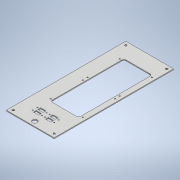
# Autodesk Inventor part: top_panel2
Saved by Autodesk Inventor 2022 (Build 260153000, 153)
## iProperties
Created: 2021-05-16
Part Number: top_panel2
Material: Generic
Document SubType Name: Modeling
Designer: gisen
Density: 1 g/cm^3
Appearance: Default
Author: gisen
Autodesk Inventor part; units mm, degrees
ref_plane "YZ Plane" through (0, 0, 0) normal (1, 0, 0) x (0, 1, 0)
ref_plane "XZ Plane" through (0, 0, 0) normal (0, 1, 0) x (-1, 0, 0)
ref_plane "XY Plane" through (0, 0, 0) normal (0, 0, 1) x (1, 0, 0)
sketch "Sketch1" plane through (0, 0, 0) normal (0, 0, 1) x (1, 0, 0)
  line L0 (-78, 195) -> (78, 195)
  line L1 (78, 195) -> (78, -195)
  line L2 (78, -195) -> (-78, -195)
  line L3 (-78, -195) -> (-78, 195)
  line L4 (-78, 195) -> (78, -195) construction
  line L5 (78, 195) -> (-78, -195) construction
  point P0 (0, 0)
  dimension "d1" = 156
  dimension "d2" = 390
  constraints: 12 end point, 2 midpoint, 2 parallel, 1 horizontal, 1 perpendicular
  measures "d1" distance of L0.start L0.end
  measures "d2" distance of L0.end L1.end
extrude "Extrusion1" add sketch "Sketch1" along normal blind 3
sketch "Sketch2" plane through (0, 0, 3) normal (0, 0, 1) x (1, 0, 0)
  line L0 (-78, -195) -> (78, -195) projected
  line L1 (-78, 195) -> (-78, -195) projected
  arc A0 (-64.4298, -185.2577) -> (-68.2577, -181.4298) centre (-66, -183) ccw
  arc A1 (-69.8472, -183.7153) -> (-66.7153, -186.8472) centre (-68, -185) ccw
  line L2 (-66.7153, -186.8472) -> (-64.4298, -185.2577)
  line L3 (-69.8472, -183.7153) -> (-68.2577, -181.4298)
  line L4 (0, 16.0888) -> (0, -25.3045)
  line L5 (-19.6832, 0) -> (22.709, 0)
  arc A2 (68.2577, -181.4298) -> (64.4298, -185.2577) centre (66, -183) ccw
  arc A3 (66.7153, -186.8472) -> (69.8472, -183.7153) centre (68, -185) ccw
  line L6 (66.7153, -186.8472) -> (64.4298, -185.2577)
  line L7 (69.8472, -183.7153) -> (68.2577, -181.4298)
  arc A4 (-68.2577, 181.4298) -> (-64.4298, 185.2577) centre (-66, 183) ccw
  arc A5 (-66.7153, 186.8472) -> (-69.8472, 183.7153) centre (-68, 185) ccw
  line L8 (-66.7153, 186.8472) -> (-64.4298, 185.2577)
  line L9 (-69.8472, 183.7153) -> (-68.2577, 181.4298)
  arc A6 (64.4298, 185.2577) -> (68.2577, 181.4298) centre (66, 183) ccw
  arc A7 (69.8472, 183.7153) -> (66.7153, 186.8472) centre (68, 185) ccw
  line L10 (66.7153, 186.8472) -> (64.4298, 185.2577)
  line L11 (69.8472, 183.7153) -> (68.2577, 181.4298)
  point P0 (0, 0)
  dimension "d11" = 12
  dimension "d12" = 10
  dimension "d13" = 12
  dimension "d14" = 10
  dimension "d15" = 5.5
  dimension "d16" = 4.5
  constraints: 24 symmetric about line, 20 end point, 16 point on circle, 8 centre point, 8 coincident, 4 tangent, 1 horizontal, 1 vertical, 6 other
  measures "d11" distance from line of L0 point (-66, -183)
  measures "d12" distance from line of L0 point (-68, -185)
  measures "d13" distance from line of L1 point (-66, -183)
  measures "d14" distance from line of L1 point (-68, -185)
  measures "d15" diameter of A0
  measures "d16" diameter of A1
extrude "Extrusion2" cut sketch "Sketch2" against normal up to surface (3 mm away)
sketch "Sketch4" plane through (0, 0, 3) normal (0, 0, 1) x (1, 0, 0)
  line L0 (-28.5, -132.4667) -> (-11.5, -132.4667)
  line L1 (-11.5, -132.4667) -> (-11.5, -141.4667)
  line L2 (-11.5, -141.4667) -> (-28.5, -141.4667)
  line L3 (-28.5, -141.4667) -> (-28.5, -132.4667)
  line L4 (-28.5, -132.4667) -> (-11.5, -141.4667) construction
  line L5 (-11.5, -132.4667) -> (-28.5, -141.4667) construction
  circle A0 centre (-35, -136.9667) radius 1.65
  circle A1 centre (-5, -136.9667) radius 1.65
  line L6 (0, -132.1595) -> (0, -155.449)
  line L7 (28.5, -132.4667) -> (11.5, -132.4667)
  line L8 (11.5, -132.4667) -> (11.5, -141.4667)
  line L9 (11.5, -141.4667) -> (28.5, -141.4667)
  line L10 (28.5, -141.4667) -> (28.5, -132.4667)
  line L11 (28.5, -132.4667) -> (11.5, -141.4667) construction
  line L12 (11.5, -132.4667) -> (28.5, -141.4667) construction
  circle A2 centre (35, -136.9667) radius 1.65
  circle A3 centre (5, -136.9667) radius 1.65
  line L13 (-30.7879, -144.4667) -> (-3.35, -144.4667)
  line L14 (-28.5, -156.4667) -> (-11.5, -156.4667)
  line L15 (-11.5, -156.4667) -> (-11.5, -147.4667)
  line L16 (-11.5, -147.4667) -> (-28.5, -147.4667)
  line L17 (-28.5, -147.4667) -> (-28.5, -156.4667)
  line L18 (-28.5, -156.4667) -> (-11.5, -147.4667) construction
  line L19 (-11.5, -156.4667) -> (-28.5, -147.4667) construction
  circle A4 centre (-35, -151.9667) radius 1.65
  circle A5 centre (-5, -151.9667) radius 1.65
  line L20 (28.5, -156.4667) -> (11.5, -156.4667)
  line L21 (11.5, -156.4667) -> (11.5, -147.4667)
  line L22 (11.5, -147.4667) -> (28.5, -147.4667)
  line L23 (28.5, -147.4667) -> (28.5, -156.4667)
  line L24 (28.5, -156.4667) -> (11.5, -147.4667) construction
  line L25 (11.5, -156.4667) -> (28.5, -147.4667) construction
  circle A6 centre (35, -151.9667) radius 1.65
  circle A7 centre (5, -151.9667) radius 1.65
  line L26 (-66.7153, 186.8472) -> (-64.4298, 185.2577) projected
  arc A8 (-68.2577, 181.4298) -> (-64.4298, 185.2577) centre (-66, 183) ccw projected
  line L27 (-68.2577, 181.4298) -> (-69.8472, 183.7153) projected
  arc A9 (-66.7153, 186.8472) -> (-69.8472, 183.7153) centre (-68, 185) ccw projected
  arc A10 (69.8472, 183.7153) -> (66.7153, 186.8472) centre (68, 185) ccw projected
  line L28 (69.8472, 183.7153) -> (68.2577, 181.4298) projected
  arc A11 (64.4298, 185.2577) -> (68.2577, 181.4298) centre (66, 183) ccw projected
  line L29 (64.4298, 185.2577) -> (66.7153, 186.8472) projected
  line L30 (66.7153, -186.8472) -> (64.4298, -185.2577) projected
  arc A12 (68.2577, -181.4298) -> (64.4298, -185.2577) centre (66, -183) ccw projected
  line L31 (68.2577, -181.4298) -> (69.8472, -183.7153) projected
  arc A13 (66.7153, -186.8472) -> (69.8472, -183.7153) centre (68, -185) ccw projected
  arc A14 (-69.8472, -183.7153) -> (-66.7153, -186.8472) centre (-68, -185) ccw projected
  line L32 (-69.8472, -183.7153) -> (-68.2577, -181.4298) projected
  arc A15 (-64.4298, -185.2577) -> (-68.2577, -181.4298) centre (-66, -183) ccw projected
  line L33 (-64.4298, -185.2577) -> (-66.7153, -186.8472) projected
  line L34 (78, 195) -> (-78, 195) projected
  line L35 (-78, 195) -> (-78, -195) projected
  line L36 (-78, -195) -> (78, -195) projected
  line L37 (78, -195) -> (78, 195) projected
  line L38 (78, -195) -> (-78, -195) projected
  point P0 (0, 0)
  point P1 (-20, -136.9667)
  point P2 (-5, -136.9667)
  point P3 (20, -136.9667)
  point P4 (-20, -151.9667)
  point P5 (20, -151.9667)
  point P6 (0, -195)
  dimension "d37" = 17
  dimension "d38" = 9
  dimension "d39" = 6.5
  dimension "d40" = 4.5
  dimension "d41" = 3.3
  dimension "d42" = 6.5
  dimension "d43" = 4.5
  dimension "d44" = 3.3
  dimension "d45" = 5
  dimension "d46" = 3
  dimension "d55" = 0
  constraints: 52 end point, 27 symmetric about line, 9 midpoint, 8 centre point, 8 coincident, 2 horizontal, 2 parallel, 1 perpendicular, 1 vertical, 6 other
  measures "d37" distance of L1.end L2.end
  measures "d38" distance of L0.end L1.end
  measures "d39" distance from line of L3 point (-35, -136.967)
  measures "d40" distance from line of point (-35, -136.967) L0
  measures "d41" diameter of A0
  measures "d42" distance from line of point (-5, -136.967) L1
  measures "d43" distance from line of L0 point (-5, -136.967)
  measures "d44" diameter of A1
  measures "d45" horizontal distance of A1.centre point (0, 0)
  measures "d46" distance between parallel lines of L13 L2
  measures "d55" distance from line of point (0, -195) L6
extrude "Extrusion4" cut sketch "Sketch4" against normal up to surface (3 mm away) contours L0 L1 L2 L3 | A0 | A1 | L10 L9 L8 L7 | A2 | A3 | L17 L16 L15 L14 | A4 | A5 | L20 L21 L22 L23 | A6 | A7
sketch "Sketch5" plane through (0, 0, 3) normal (0, 0, 1) x (1, 0, 0)
  line L0 (-78, -195) -> (78, -195) projected
  line L1 (-2.4755, -172.54) -> (2.4755, -172.54)
  line L2 (-2.4755, -187.46) -> (2.4755, -187.46)
  arc A0 (-2.4755, -172.54) -> (-2.4755, -187.46) centre (0, -180) ccw
  arc A1 (2.4755, -187.46) -> (2.4755, -172.54) centre (0, -180) ccw
  point P0 (0, 0)
  dimension "d49" = 15
  dimension "d51" = 7.46
  dimension "d52" = 7.46
  constraints: 4 end point, 4 point on circle, 2 centre point, 2 horizontal, 1 coincident
  measures "d49" distance from line of L0 point (0, -180)
  measures "d51" distance from line of A0.centre L1
  measures "d52" distance from line of point (0, -180) L2
extrude "Extrusion5" cut sketch "Sketch5" against normal up to surface (3 mm away)
sketch "Sketch7" plane through (0, 0, 3) normal (0, 0, 1) x (1, 0, 0)
  circle A0 centre (-38, -90.5) radius 2
  line L0 (-2.4755, -172.54) -> (2.4755, -172.54) projected
  arc A1 (2.4755, -187.46) -> (2.4755, -172.54) centre (0, -180) ccw projected
  line L1 (2.4755, -187.46) -> (-2.4755, -187.46) projected
  arc A2 (-2.4755, -172.54) -> (-2.4755, -187.46) centre (0, -180) ccw projected
  line L2 (-11.5, -156.4667) -> (-28.5, -156.4667) projected
  line L3 (-28.5, -156.4667) -> (-28.5, -147.4667) projected
  line L4 (-28.5, -147.4667) -> (-11.5, -147.4667) projected
  line L5 (-11.5, -147.4667) -> (-11.5, -156.4667) projected
  line L6 (11.5, -147.4667) -> (28.5, -147.4667) projected
  line L7 (28.5, -147.4667) -> (28.5, -156.4667) projected
  line L8 (28.5, -156.4667) -> (11.5, -156.4667) projected
  line L9 (11.5, -156.4667) -> (11.5, -147.4667) projected
  line L10 (11.5, -132.4667) -> (28.5, -132.4667) projected
  line L11 (28.5, -132.4667) -> (28.5, -141.4667) projected
  line L12 (28.5, -141.4667) -> (11.5, -141.4667) projected
  line L13 (11.5, -141.4667) -> (11.5, -132.4667) projected
  circle A3 centre (35, -151.9667) radius 1.65 projected
  circle A4 centre (-35, -151.9667) radius 1.65 projected
  circle A5 centre (5, -136.9667) radius 1.65 projected
  circle A6 centre (-5, -136.9667) radius 1.65 projected
  circle A7 centre (-35, -136.9667) radius 1.65 projected
  circle A8 centre (35, -136.9667) radius 1.65 projected
  circle A9 centre (-5, -151.9667) radius 1.65 projected
  circle A10 centre (5, -151.9667) radius 1.65 projected
  line L14 (-11.5, -132.4667) -> (-11.5, -141.4667) projected
  line L15 (-11.5, -141.4667) -> (-28.5, -141.4667) projected
  line L16 (-28.5, -141.4667) -> (-28.5, -132.4667) projected
  line L17 (-28.5, -132.4667) -> (-11.5, -132.4667) projected
  line L18 (-66.7153, 186.8472) -> (-64.4298, 185.2577) projected
  arc A11 (-68.2577, 181.4298) -> (-64.4298, 185.2577) centre (-66, 183) ccw projected
  line L19 (-68.2577, 181.4298) -> (-69.8472, 183.7153) projected
  arc A12 (-66.7153, 186.8472) -> (-69.8472, 183.7153) centre (-68, 185) ccw projected
  arc A13 (69.8472, 183.7153) -> (66.7153, 186.8472) centre (68, 185) ccw projected
  line L20 (69.8472, 183.7153) -> (68.2577, 181.4298) projected
  arc A14 (64.4298, 185.2577) -> (68.2577, 181.4298) centre (66, 183) ccw projected
  line L21 (64.4298, 185.2577) -> (66.7153, 186.8472) projected
  line L22 (66.7153, -186.8472) -> (64.4298, -185.2577) projected
  arc A15 (68.2577, -181.4298) -> (64.4298, -185.2577) centre (66, -183) ccw projected
  line L23 (68.2577, -181.4298) -> (69.8472, -183.7153) projected
  arc A16 (66.7153, -186.8472) -> (69.8472, -183.7153) centre (68, -185) ccw projected
  arc A17 (-69.8472, -183.7153) -> (-66.7153, -186.8472) centre (-68, -185) ccw projected
  line L24 (-69.8472, -183.7153) -> (-68.2577, -181.4298) projected
  arc A18 (-64.4298, -185.2577) -> (-68.2577, -181.4298) centre (-66, -183) ccw projected
  line L25 (-64.4298, -185.2577) -> (-66.7153, -186.8472) projected
  line L26 (78, 195) -> (-78, 195) projected
  line L27 (-78, 195) -> (-78, -195) projected
  line L28 (-78, -195) -> (78, -195) projected
  line L29 (78, -195) -> (78, 195) projected
  circle A19 centre (-38, 14.5) radius 2
  circle A20 centre (-38, 30) radius 2
  circle A21 centre (-38, 135) radius 2
  line L30 (14.5, 19.3358) -> (14.5, -21.6)
  circle A22 centre (67, -90.5) radius 2
  circle A23 centre (67, 14.5) radius 2
  circle A24 centre (67, 30) radius 2
  circle A25 centre (67, 135) radius 2
  point P0 (0, 0)
  dimension "d56" = 4
  dimension "d57" = 40
  dimension "d60" = 4
  dimension "d61" = 105
  dimension "d62" = 40
  dimension "d63" = 4
  dimension "d65" = 40
  dimension "d66" = 4
  dimension "d68" = 40
  dimension "d69" = 60
  dimension "d103" = 15.5
  dimension "d104" = 105
  dimension "d112" = 52.5
  constraints: 8 centre point, 4 symmetric about line, 2 end point, 1 vertical, 4 other
  measures "d56" diameter of A0
  measures "d57" distance from line of L27 A0.centre
  measures "d60" diameter of A19
  measures "d61" distance of A0.centre A19.centre
  measures "d62" distance from line of L27 A19.centre
  measures "d63" diameter of A20
  measures "d65" distance from line of L27 A20.centre
  measures "d66" diameter of A21
  measures "d68" distance from line of L27 A21.centre
  measures "d69" distance from line of L26 A21.centre
  measures "d103" distance of A19.centre A20.centre
  measures "d104" distance of A21.centre A20.centre
  measures "d112" distance from line of A19.centre L30
extrude "Extrusion7" cut sketch "Sketch7" against normal up to surface (3 mm away) contours A0 | A19 | A20 | A21 | A22 | A23 | A24 | A25
sketch "Sketch8" plane through (0, 0, 3) normal (0, 0, 1) x (1, 0, 0)
  circle A0 centre (-38, -90.5) radius 2 projected
  circle A1 centre (-38, 14.5) radius 2 projected
  circle A2 centre (67, 30) radius 2 projected
  circle A3 centre (67, 135) radius 2 projected
  circle A4 centre (67, -90.5) radius 2 projected
  circle A5 centre (67, 14.5) radius 2 projected
  circle A6 centre (-38, 30) radius 2 projected
  circle A7 centre (-38, 135) radius 2 projected
  line L0 (-2.4755, -172.54) -> (2.4755, -172.54) projected
  arc A8 (2.4755, -187.46) -> (2.4755, -172.54) centre (0, -180) ccw projected
  line L1 (2.4755, -187.46) -> (-2.4755, -187.46) projected
  arc A9 (-2.4755, -172.54) -> (-2.4755, -187.46) centre (0, -180) ccw projected
  line L2 (-11.5, -156.4667) -> (-28.5, -156.4667) projected
  line L3 (-28.5, -156.4667) -> (-28.5, -147.4667) projected
  line L4 (-28.5, -147.4667) -> (-11.5, -147.4667) projected
  line L5 (-11.5, -147.4667) -> (-11.5, -156.4667) projected
  line L6 (11.5, -147.4667) -> (28.5, -147.4667) projected
  line L7 (28.5, -147.4667) -> (28.5, -156.4667) projected
  line L8 (28.5, -156.4667) -> (11.5, -156.4667) projected
  line L9 (11.5, -156.4667) -> (11.5, -147.4667) projected
  line L10 (11.5, -132.4667) -> (28.5, -132.4667) projected
  line L11 (28.5, -132.4667) -> (28.5, -141.4667) projected
  line L12 (28.5, -141.4667) -> (11.5, -141.4667) projected
  line L13 (11.5, -141.4667) -> (11.5, -132.4667) projected
  circle A10 centre (35, -151.9667) radius 1.65 projected
  circle A11 centre (-35, -151.9667) radius 1.65 projected
  circle A12 centre (5, -136.9667) radius 1.65 projected
  circle A13 centre (-5, -136.9667) radius 1.65 projected
  circle A14 centre (-35, -136.9667) radius 1.65 projected
  circle A15 centre (35, -136.9667) radius 1.65 projected
  circle A16 centre (-5, -151.9667) radius 1.65 projected
  circle A17 centre (5, -151.9667) radius 1.65 projected
  line L14 (-11.5, -132.4667) -> (-11.5, -141.4667) projected
  line L15 (-11.5, -141.4667) -> (-28.5, -141.4667) projected
  line L16 (-28.5, -141.4667) -> (-28.5, -132.4667) projected
  line L17 (-28.5, -132.4667) -> (-11.5, -132.4667) projected
  line L18 (-66.7153, 186.8472) -> (-64.4298, 185.2577) projected
  arc A18 (-68.2577, 181.4298) -> (-64.4298, 185.2577) centre (-66, 183) ccw projected
  line L19 (-68.2577, 181.4298) -> (-69.8472, 183.7153) projected
  arc A19 (-66.7153, 186.8472) -> (-69.8472, 183.7153) centre (-68, 185) ccw projected
  arc A20 (69.8472, 183.7153) -> (66.7153, 186.8472) centre (68, 185) ccw projected
  line L20 (69.8472, 183.7153) -> (68.2577, 181.4298) projected
  arc A21 (64.4298, 185.2577) -> (68.2577, 181.4298) centre (66, 183) ccw projected
  line L21 (64.4298, 185.2577) -> (66.7153, 186.8472) projected
  line L22 (66.7153, -186.8472) -> (64.4298, -185.2577) projected
  arc A22 (68.2577, -181.4298) -> (64.4298, -185.2577) centre (66, -183) ccw projected
  line L23 (68.2577, -181.4298) -> (69.8472, -183.7153) projected
  arc A23 (66.7153, -186.8472) -> (69.8472, -183.7153) centre (68, -185) ccw projected
  arc A24 (-69.8472, -183.7153) -> (-66.7153, -186.8472) centre (-68, -185) ccw projected
  line L24 (-69.8472, -183.7153) -> (-68.2577, -181.4298) projected
  arc A25 (-64.4298, -185.2577) -> (-68.2577, -181.4298) centre (-66, -183) ccw projected
  line L25 (-64.4298, -185.2577) -> (-66.7153, -186.8472) projected
  line L26 (78, 195) -> (-78, 195) projected
  line L27 (-78, 195) -> (-78, -195) projected
  line L28 (-78, -195) -> (78, -195) projected
  line L29 (78, -195) -> (78, 195) projected
  circle A26 centre (-38, 135) radius 2 projected
  circle A27 centre (-38, 135) radius 6.33
  line L30 (-31.67, 135) -> (-31.67, 13.6115)
  arc A28 (-24.17, 142.5) -> (-31.67, 135) centre (-24.17, 135) ccw
  line L31 (-31.67, 13.6115) -> (-31.67, -90.5)
  arc A29 (-31.67, -90.5) -> (-24.17, -98) centre (-24.17, -90.5) ccw
  line L32 (-24.17, -98) -> (-10.2337, -98)
  line L33 (-24.17, 142.5) -> (-11.5, 142.5)
  line L34 (14.5, 11.7665) -> (14.5, -13.3152)
  line L35 (60.67, 135) -> (60.67, 13.6115)
  arc A30 (60.67, 135) -> (53.17, 142.5) centre (53.17, 135) ccw
  line L36 (60.67, 13.6115) -> (60.67, -90.5)
  arc A31 (53.17, -98) -> (60.67, -90.5) centre (53.17, -90.5) ccw
  line L37 (53.17, -98) -> (39.2337, -98)
  line L38 (53.17, 142.5) -> (40.5, 142.5)
  line L39 (40.5, 142.5) -> (-11.5, 142.5)
  line L40 (39.2337, -98) -> (12.6121, -98)
  circle A32 centre (-38, -90.5) radius 2 projected
  line L41 (-10.2337, -98) -> (21.6365, -98)
  point P0 (0, 0)
  point P1 (14.5, 82.5)
  point P2 (14.5, -38)
  point P3 (3.676, -78)
  point P4 (12.6121, -98)
  dimension "d90" = 52.5
  dimension "d91" = 52.5
  dimension "d94" = 7.5
  dimension "d96" = 52.5
  dimension "d97" = 52.5
  dimension "d100" = 7.5
  dimension "d107" = 60
  dimension "d108" = 60
  dimension "d109" = 7.5
  dimension "d113" = 52.5
  constraints: 24 end point, 9 symmetric about line, 8 point on circle, 4 centre point, 4 point on line, 3 horizontal, 3 tangent, 3 vertical, 2 coincident, 1 horizontal alignment, 1 perpendicular, 4 other
  measures "d90" horizontal distance of A7.centre point (14.5, 82.5)
  measures "d91" horizontal distance of A7.centre point (14.5, 82.5)
  measures "d94" radius of A28
  measures "d96" horizontal distance of A0.centre point (14.5, -38)
  measures "d97" horizontal distance of point (14.5, -38) A0.centre
  measures "d100" distance from line of L31 point (-24.17, -90.5)
  measures "d107" distance from line of point (14.5, 82.5) L39
  measures "d108" distance from line of point (14.5, -38) L37
  measures "d109" distance from line of L32 A29.centre
  measures "d113" distance from line of A1.centre L34
extrude "Extrusion9" cut sketch "Sketch8" against normal up to surface (3 mm away) contours A28 L33 L39 L38 A30 L35 L36 A31 L37 L40 L41 L32 A29 L31 L30
equation "\"d13\" = d11"
equation "\"d14\" = d12"
equation "\"d42\" = d39"
equation "\"d44\" = d41"
equation "\"d62\" = d57"
equation "\"d65\" = d62"
equation "\"d68\" = d65"
equation "\"d104\" = d61"
equation "\"d87\" = d62"
equation "\"d91\" = d90"
equation "\"d97\" = d96"
equation "\"d100\" = d99"
equation "\"d109\" = d100"
equation "\"d26\" = d24"
equation "\"d28\" = d26"
equation "\"d99\" = d95"
equation "\"d24\" = 44.7"
equation "\"d95\" = 7.5"
body "Solid1"
